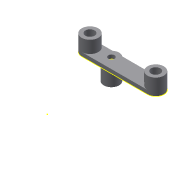
# Autodesk Inventor part: palm_board_frame
Saved by Autodesk Inventor 2014 (Build 180170000, 170)
## iProperties
Created: 2015-08-26
Part Number: palm_board_frame
Material: Generic
Document SubType Name: Modeling
Designer: Martin
Density: 1 g/cm^3
Appearance: Default
Author: Martin
Autodesk Inventor part; units mm, degrees
note: some values were not read from the file. Chosen so that the rebuilt part matches the saved one: sketch regions of "Extrusion1".
sketch "Sketch1" plane through (0, 0, 0) normal (0, 0, 1) x (1, 0, 0)
  circle A0 centre (-40.6954, 81.5546) radius 2.65 projected
  circle A1 centre (-40.6954, 81.5546) radius 1 projected
  circle A2 centre (-10.6954, 24.5546) radius 2.6954 projected
  circle A3 centre (-10.6954, 24.5546) radius 1 projected
  line L0 (-44.1736, 21.5546) -> (-0.6736, 21.5546) construction
  line L1 (-0.6736, 21.5546) -> (-0.6736, 80.0546) construction
  line L2 (-0.6736, 80.0546) -> (-44.1736, 80.0546) construction
  line L3 (-44.1736, 80.0546) -> (-44.1736, 21.5546) construction
  circle A4 centre (-40.6954, 81.5546) radius 1.5 construction
  line L4 (1.3264, 150.3987) -> (1.3264, -151.5753) construction
  circle A5 centre (-4.4736, 25.3046) radius 0.95 construction
  line L5 (-4.4736, 24.3546) -> (-4.4736, 21.5546) construction
  line L6 (-3.5236, 25.3046) -> (-0.6736, 25.3046) construction
  circle A6 centre (-4.4736, 25.3046) radius 1
  circle A7 centre (10.6566, 24.5546) radius 2.6566 projected
  circle A8 centre (10.6566, 24.5546) radius 1 projected
  line L7 (-10.6905, 27.25) -> (10.6614, 27.2112)
  line L8 (10.6614, 21.8981) -> (-10.6905, 21.8593)
  arc A9 (-10.6905, 27.25) -> (-10.6905, 21.8593) centre (-10.6954, 24.5546) ccw
  arc A10 (10.6614, 21.8981) -> (10.6614, 27.2112) centre (10.6566, 24.5546) ccw
  circle A11 centre (-4.4736, 25.3046) radius 2.5
  circle A12 centre (-10.6954, 24.5546) radius 2.6954
  circle A13 centre (10.6566, 24.5546) radius 2.6566
  point P0 (0, 0)
  dimension "d0" = 58.5
  dimension "d1" = 43.5
  dimension "d2" = 3
  dimension "d3" = 2
  dimension "d4" = 1.9
  dimension "d5" = 2.8
  dimension "d6" = 2.85
  dimension "d7" = 2
  dimension "d8" = 5
  constraints: 18 end point, 10 point on circle, 9 tangent, 6 centre point, 5 coincident, 4 point on line, 2 parallel, 2 perpendicular, 1 horizontal, 1 vertical, 8 other
  measures "d0" distance of L2.end L0.start
  measures "d1" distance of L0.start L0.end
  measures "d2" diameter of A4
  measures "d3" distance between parallel lines of L4 L1
  measures "d4" diameter of A5
  measures "d5" distance of L5.start L5.end
  measures "d6" distance of L6.start L6.end
  measures "d7" diameter of A6
  measures "d8" diameter of A11
ref_plane "Work Plane1" through (0, 0, 3.75) normal (0, 0, 1) x (1, 0, 0)
ref_plane "Work Plane2" through (-7.5, 22.75, 5) normal (0, 0, -1) x (0, 1, 0)
extrude "Extrusion1" add sketch "Sketch1" along normal up to surface (1.25 mm away) from surface at 3.75 contours A2 | A2 L7 A11 A7 L8 | A11 L7 | L7 A11 | A7
sketch "Sketch2" plane through (-10.6954, 24.5546, 5) normal (0, 0, 1) x (1, 0, 0)
  circle A0 centre (0, 0) radius 1 projected
  circle A1 centre (21.352, 0) radius 1 projected
  arc A2 (21.3568, -2.6566) -> (21.3568, 2.6566) centre (21.352, 0) ccw projected
  arc A3 (0.0049, 2.6954) -> (0.0049, -2.6954) centre (0, 0) ccw projected
  circle A4 centre (21.352, 0) radius 2.6566
  circle A5 centre (0, 0) radius 2.6954
  point P0 (10.6954, -24.5546)
  constraints: 2 centre point, 2 coincident, 2 concentric
ref_plane "Work Plane3" through (-13.3907, 21.8593, 8) normal (0, 0, -1) x (0, 1, 0)
sketch "Sketch3" plane through (-10.6954, 24.5546, 3.75) normal (0, 0, -1) x (-1, 0, 0)
  circle A0 centre (0, 0) radius 1 projected
  circle A1 centre (-21.352, 0) radius 1 projected
  circle A2 centre (-6.2217, 0.75) radius 1 projected
  line L0 (-21.3568, -2.6566) -> (-0.0049, -2.6954) projected
  arc A3 (-0.0049, -2.6954) -> (-0.0049, 2.6954) centre (0, 0) ccw projected
  line L1 (-0.0049, 2.6954) -> (-4.6411, 2.6869) projected
  arc A4 (-4.6411, 2.6869) -> (-7.8093, 2.6812) centre (-6.2217, 0.75) ccw projected
  line L2 (-7.8093, 2.6812) -> (-21.3568, 2.6566) projected
  arc A5 (-21.3568, 2.6566) -> (-21.3568, -2.6566) centre (-21.352, 0) ccw projected
  point P0 (-10.6954, -24.5546)
ref_plane "Work Plane4" through (-13.3907, 21.8593, 8) normal (0, 0, -1) x (0, 1, 0)
extrude "Extrusion3" add sketch "Sketch2" along normal blind 4
sketch "Sketch4" plane through (-10.6954, 24.5546, 3.75) normal (0, 0, -1) x (-1, 0, 0)
  circle A0 centre (-6.2217, 0.75) radius 1 projected
  arc A1 (-4.6411, 2.6869) -> (-7.8093, 2.6812) centre (-6.2217, 0.75) ccw projected
  circle A2 centre (-6.2217, 0.75) radius 2.5
  point P0 (-10.6954, -24.5546)
  constraints: 1 centre point, 1 coincident
extrude "Extrusion4" add sketch "Sketch4" along normal blind 5.5
chamfer "Chamfer1" distance 1 angle 45 1 edges at (-4.4691, 27.8046, 3.75)
sketch "Sketch5" plane through (0, 0, 0) normal (0, 0, 1) x (1, 0, 0)
  circle A0 centre (10.6566, 24.5546) radius 1 projected
  circle A1 centre (-4.4736, 25.3046) radius 1 projected
  circle A2 centre (-10.6954, 24.5546) radius 1 projected
  circle A3 centre (-10.6954, 24.5546) radius 1.5
  circle A4 centre (10.6566, 24.5546) radius 1.5
  point P0 (0, 0)
  dimension "d21" = 3
  dimension "d22" = 3
  constraints: 2 centre point, 2 coincident
  measures "d21" diameter of A3
  measures "d22" diameter of A4
extrude "Extrusion5" cut sketch "Sketch5" along normal through all contours A0 | A2 | A3 | A4
body "Solid1"
